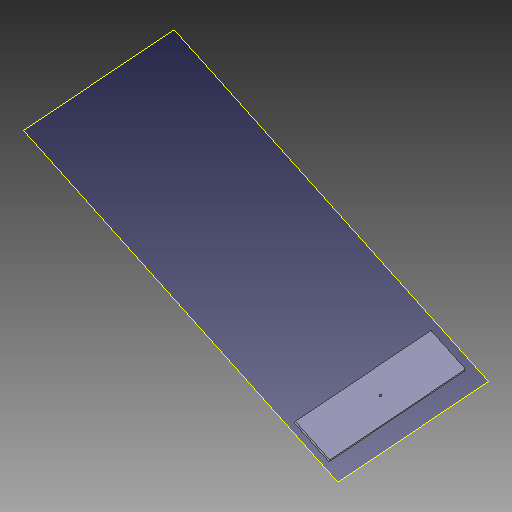
# Autodesk Inventor part: Fram
Saved by Autodesk Inventor 2019 (Build 230136000, 136)
## iProperties
Created: 2018-12-19
Part Number: Fram
Material: Generic
Document SubType Name: Modeling
Designer: Filip
Density: 1 g/cm^3
Appearance: Default
Author: Filip
Autodesk Inventor part; units mm, degrees
ref_plane "YZ Plane" through (0, 0, 0) normal (1, 0, 0) x (0, 1, 0)
ref_plane "XZ Plane" through (0, 0, 0) normal (0, 1, 0) x (-1, 0, 0)
ref_plane "XY Plane" through (0, 0, 0) normal (0, 0, 1) x (1, 0, 0)
ref_plane "Work Plane1" through (-728.8112, -105.3847, 288.112) normal (-0.4570507, -0.8833415, -0.1039826) x (0.88913, -0.4568478, -0.0271666)
sketch "Sketch1" plane through (-728.8112, -105.3847, 288.112) normal (-0.4570507, -0.8833415, -0.1039826) x (0.88913, -0.4568478, -0.0271666)
  line L0 (-49.7406, -45) -> (-49.7406, -53)
  line L1 (-49.7406, -53) -> (123, -53)
  line L2 (123, -53) -> (123, 53)
  line L3 (123, 53) -> (-49.7406, 53)
  line L4 (-49.7406, 53) -> (-49.7406, 45)
  line L5 (-49.7406, 45) -> (-91.8594, 45)
  line L6 (-91.8594, 45) -> (-91.8594, 53)
  line L7 (-91.8594, 53) -> (-123, 53)
  line L8 (-123, 53) -> (-123, -53)
  line L9 (-123, -53) -> (-91.8594, -53)
  line L10 (-91.8594, -53) -> (-91.8594, -45)
  line L11 (-91.8594, -45) -> (-49.7406, -45)
  line L12 (-95.4, -15.0028) -> (-111.4, -15.0028)
  line L13 (-111.4, -15.0028) -> (-111.4, 13.9972)
  line L14 (-111.4, 13.9972) -> (-95.4, 13.9972)
  line L15 (-95.4, 13.9972) -> (-95.4, -15.0028)
  line L16 (123, 53) -> (93, 53)
  line L17 (93, 53) -> (93, -53)
  line L18 (93, -53) -> (123, -53)
  line L19 (123, -53) -> (123, 53)
  point P0 (607.6902, -314.6271)
  dimension "d0" = 30
  constraints: 40 end point, 2 parallel, 1 horizontal, 1 perpendicular, 1 point on line
  measures "d0" distance between parallel lines of L2 L17
extrude "Extrusion1" add sketch "Sketch1" along normal blind 2 contours L17 L3 L2 L1
sketch "Sketch4" plane through (-729.7253, -107.1513, 287.9041) normal (-0.4570507, -0.8833415, -0.1039826) x (0.88913, -0.4568478, -0.0271666)
  circle A0 centre (108, 0) radius 0.85
  point P0 (607.6902, -314.6271)
  constraints: 1 centre point
extrude "Extrusion4" cut sketch "Sketch4" against normal up to next
thread "Thread1" size "M1.7x0.35" class "6H" standard "ISO Metric profile" full length
body "Solid1"
